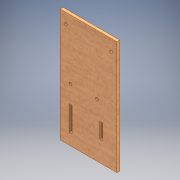
# Autodesk Inventor part: podstawa podstawa
Saved by Autodesk Inventor 2017 (Build 210142000, 142)
## iProperties
Created: 2017-05-18
Part Number: podstawa podstawa
Material: Drewno (wiśnia)
Document SubType Name: Modeling
Designer: Damian
Density: 0.63 g/cm^3
Appearance: Wiśnia — naturalna — niski połysk
Author: Damian
Autodesk Inventor part; units mm, degrees
ref_plane "YZ Plane" through (0, 0, 0) normal (1, 0, 0) x (0, 1, 0)
ref_plane "XZ Plane" through (0, 0, 0) normal (0, 1, 0) x (-1, 0, 0)
ref_plane "XY Plane" through (0, 0, 0) normal (0, 0, 1) x (1, 0, 0)
sketch "Szkic1" plane through (0, 0, 0) normal (0, 1, 0) x (-1, 0, 0)
  line L0 (0, 0) -> (60, 0)
  line L1 (60, 0) -> (60, -120)
  line L2 (60, -120) -> (0, -120)
  line L3 (0, -120) -> (0, 0)
  line L4 (50.5, -108) -> (47.5, -108)
  line L5 (47.5, -108) -> (47.5, -82)
  line L6 (47.5, -82) -> (50.5, -82)
  line L7 (50.5, -82) -> (50.5, -108)
  line L8 (15, -82) -> (18, -82)
  line L9 (18, -82) -> (18, -98)
  line L10 (18, -98) -> (15, -98)
  line L11 (15, -98) -> (15, -82)
  dimension "d0" = 60
  dimension "d1" = 120
  dimension "d2" = 3
  dimension "d3" = 26
  dimension "d4" = 12
  dimension "d5" = 9.5
  dimension "d6" = 3
  dimension "d7" = 16
  dimension "d9" = 22
  dimension "d26" = 29.5
  constraints: 24 end point, 6 parallel, 3 horizontal, 3 perpendicular
  measures "d0" distance of L1.end L2.end
  measures "d1" distance of L0.end L1.end
  measures "d2" distance of L5.end L6.end
  measures "d3" distance of L4.end L5.end
  measures "d4" distance between parallel lines of L2 L4
  measures "d5" distance between parallel lines of L1 L7
  measures "d6" distance of L9.end L10.end
  measures "d7" distance of L8.end L9.end
  measures "d9" distance between parallel lines of L2 L10
  measures "d26" distance between parallel lines of L5 L9
extrude "Wyciągnięcie proste1" add sketch "Szkic1" along normal blind 3
sketch "Szkic2" plane through (0, 0, 0) normal (0, -1, 0) x (1, 0, 0)
  line L0 (-50.5, -82) -> (-47.5, -82) projected
  line L1 (-60, 0) -> (-60, -120) projected
  point P0 (0, 0)
  point P1 (-49, -63)
  point P2 (-21.1, -63)
  point P3 (-6, -12.2)
  point P4 (-54.1, -10.9)
  dimension "d12" = 19
  dimension "d13" = 11
  dimension "d14" = 27.9
  dimension "d15" = 50.8
  dimension "d16" = 54
  dimension "d17" = 1.3
  dimension "d18" = 5.9
  measures "d12" distance from line of point (-49, -63) L0
  measures "d13" distance from line of point (-49, -63) L1
  measures "d14" distance of point (-21.1, -63) point (-49, -63)
  measures "d15" vertical distance of point (-21.1, -63) point (-6, -12.2)
  measures "d16" distance from line of L1 point (-6, -12.2)
  measures "d17" vertical distance of point (-54.1, -10.9) point (-6, -12.2)
  measures "d18" distance from line of L1 point (-54.1, -10.9)
hole "Otwór1" at (-49, 0, -63) at (-21.1, 0, -63) at (-6, 0, -12.2) at (-54.1, 0, -10.9) direction (0, 1, 0) diameter 3 end through all
